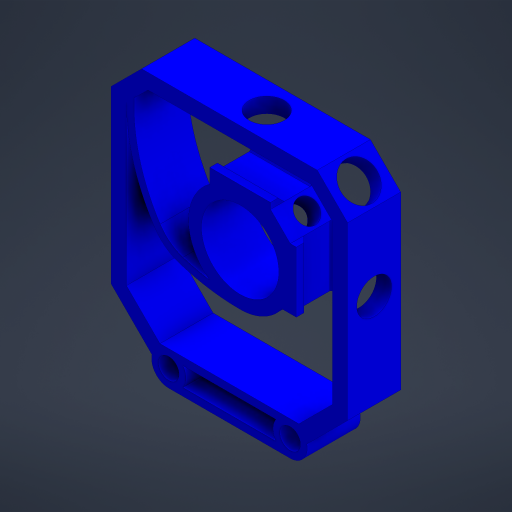
# Autodesk Inventor part: Laser Holder (Blue Laser)
Saved by Autodesk Inventor 2023.4 (Build 274418000, 418)
## iProperties
Created: 2022-07-25
Part Number: Laser Holder (Blue Laser)
Material: Generic
Document SubType Name: Modeling
Designer: xSibe
Density: 1 g/cm^3
Appearance: Plastic Blue
Author: xSibe
Autodesk Inventor part; units mm, degrees
ref_plane "YZ Plane" through (0, 0, 0) normal (1, 0, 0) x (0, 1, 0)
ref_plane "XZ Plane" through (0, 0, 0) normal (0, 1, 0) x (-1, 0, 0)
sketch "Sketch1" plane through (0, 0, 0) normal (0, 0, 1) x (1, 0, 0)
  circle A0 centre (10, 3.85) radius 1.5625
  circle A1 centre (-10, 3.85) radius 1.5625
  line L0 (-16.9, 0) -> (16.9, 0)
  line L1 (16.9, 0) -> (16.9, 7.7)
  line L2 (-16.9, 7.7) -> (16.9, 7.7)
  line L3 (-16.9, 0) -> (-16.9, 7.7)
  circle A2 centre (-10, 3.85) radius 2.8125
  circle A3 centre (10, 3.85) radius 2.8125
  line L4 (-10, 6.6625) -> (10, 6.6625)
  line L5 (10, 1.0375) -> (-10, 1.0375)
  line L6 (-10, 2.2875) -> (10, 2.2875)
  line L7 (-10, 5.4125) -> (10, 5.4125)
  line L8 (-17.05, 7.7) -> (-17.05, 42.1)
  line L9 (17.05, 7.7) -> (17.05, 42.1)
  line L10 (-17.05, 24.9) -> (17.05, 24.9)
  line L11 (0, 24.9) -> (1.767767, 26.667767)
  line L12 (0, 24.9) -> (2.5, 24.9) construction
  circle A4 centre (1.767767, 26.667767) radius 6.375
  circle A5 centre (1.767767, 26.667767) radius 5.7
  circle A6 centre (1.767767, 26.667767) radius 8.5
  line L13 (1.767767, 26.667767) -> (1.767767, 35.167767)
  line L14 (1.767767, 35.167767) -> (1.767767, 34.667767)
  line L15 (-3.232233, 33.417767) -> (6.767767, 33.417767)
  line L16 (6.767767, 33.417767) -> (6.767767, 35.917767)
  line L17 (6.767767, 35.917767) -> (-3.232233, 35.917767)
  line L18 (-3.232233, 35.917767) -> (-3.232233, 33.417767)
  line L19 (-3.232233, 33.417767) -> (6.767767, 35.917767) construction
  line L20 (6.767767, 33.417767) -> (-3.232233, 35.917767) construction
  line L21 (1.767767, 26.667767) -> (7.778175, 32.678175)
  line L22 (7.778175, 32.678175) -> (7.336233, 32.236233)
  line L23 (10.16466, 31.529126) -> (6.629126, 35.06466)
  line L24 (6.629126, 35.06466) -> (4.507806, 32.94334)
  line L25 (4.507806, 32.94334) -> (8.04334, 29.407806)
  line L26 (8.04334, 29.407806) -> (10.16466, 31.529126)
  line L27 (10.16466, 31.529126) -> (4.507806, 32.94334) construction
  line L28 (6.629126, 35.06466) -> (8.04334, 29.407806) construction
  line L29 (10.16466, 31.529126) -> (15.16466, 31.529126) construction
  line L30 (8.517767, 21.667767) -> (8.517767, 31.667767)
  line L31 (8.517767, 31.667767) -> (11.017767, 31.667767)
  line L32 (11.017767, 31.667767) -> (11.017767, 21.667767)
  line L33 (11.017767, 21.667767) -> (8.517767, 21.667767)
  line L34 (1.767767, 35.167767) -> (1.767767, 37.167767)
  line L35 (11.017767, 26.667767) -> (13.017767, 26.667767)
  line L36 (-10.217767, 5.432233) -> (10.217767, 5.432233)
  line L37 (19.467767, 14.682233) -> (19.467767, 39.367767)
  line L38 (14.467767, 44.367767) -> (-14.467767, 44.367767)
  line L39 (-19.467767, 39.367767) -> (-19.467767, 14.682233)
  line L40 (-19.467767, 5.432233) -> (19.467767, 44.367767) construction
  line L41 (19.467767, 5.432233) -> (-19.467767, 44.367767) construction
  line L42 (-10.217767, 5.432233) -> (-19.467767, 14.682233)
  line L43 (10.217767, 5.432233) -> (19.467767, 14.682233)
  line L44 (14.467767, 44.367767) -> (19.467767, 39.367767)
  line L45 (-14.467767, 44.367767) -> (-19.467767, 39.367767)
  line L46 (-15.503301, 46.867767) -> (-21.967767, 40.403301)
  line L47 (-21.967767, 40.403301) -> (-21.967767, 13.646699)
  line L48 (-21.967767, 13.646699) -> (-11.253301, 2.932233)
  line L49 (-11.253301, 2.932233) -> (11.253301, 2.932233)
  line L50 (11.253301, 2.932233) -> (21.967767, 13.646699)
  line L51 (21.967767, 13.646699) -> (21.967767, 40.403301)
  line L52 (21.967767, 40.403301) -> (15.503301, 46.867767)
  line L53 (15.503301, 46.867767) -> (-15.503301, 46.867767)
  line L54 (-13.432233, 41.867767) -> (-16.967767, 38.332233)
  line L55 (-16.967767, 38.332233) -> (-16.967767, 15.717767)
  line L56 (-16.967767, 15.717767) -> (-9.182233, 7.932233)
  line L57 (-9.182233, 7.932233) -> (9.182233, 7.932233)
  line L58 (9.182233, 7.932233) -> (16.967767, 15.717767)
  line L59 (16.967767, 15.717767) -> (16.967767, 38.332233)
  line L60 (16.967767, 38.332233) -> (13.432233, 41.867767)
  line L61 (13.432233, 41.867767) -> (-13.432233, 41.867767)
  line L62 (16.967767, 15.717767) -> (16.967767, 8.646699)
  line L63 (-16.967767, 15.717767) -> (-16.967767, 12.182233)
  line L64 (-19.467767, 14.682233) -> (-19.467767, 11.146699)
  line L65 (19.467767, 14.682233) -> (19.467767, 11.146699)
  circle A7 centre (-10, 3.85) radius 1.705
  circle A8 centre (10, 3.85) radius 1.707
  line L66 (1.767767, 18.167767) -> (-10.732233, 18.167767)
  line L67 (-10.732233, 18.167767) -> (-10.732233, 20.667767)
  arc A9 (-10.732233, 20.667767) -> (1.767767, 18.167767) centre (1.767767, 50.667767) ccw
  arc A10 (-16.967767, 38.332233) -> (-10.732233, 20.667767) centre (11.170581, 38.332233) ccw
  arc A11 (-15.687259, 39.612741) -> (-9.956996, 21.700675) centre (11.170581, 38.332233) ccw
  arc A12 (-9.956996, 21.700675) -> (-3.278671, 19.827923) centre (1.767767, 50.667767) ccw
  line L68 (-9.956996, 21.700675) -> (-11.410357, 23.734819)
  line L69 (-10.732233, 20.667767) -> (-12.213666, 22.681558)
  arc A13 (-12.213666, 22.681558) -> (-8.44317, 19.813484) centre (-6.151219, 26.73905) ccw
  arc A14 (-11.410357, 23.734819) -> (-7.660174, 20.873868) centre (-5.557613, 27.518317) ccw
  line L70 (-10, 6.6625) -> (-11.448034, 6.6625)
  line L71 (10, 6.6625) -> (11.448034, 6.6625)
  point P0 (0, 0)
  point P1 (-7.661464, 2.2875)
  point P2 (-7.661464, 5.4125)
  point P3 (7.661464, 5.4125)
  point P4 (7.661464, 2.2875)
  point P5 (7.341455, 2.932233)
  point P6 (-7.341455, 2.932233)
  point P7 (-11.185824, 6.40029)
  point P8 (11.185824, 6.40029)
  point P9 (-3.232233, 33.54163)
  point P10 (8.64163, 21.667767)
  point P11 (8.64163, 31.667767)
  point P12 (9.280097, 30.644563)
  point P13 (5.744563, 34.180097)
  point P14 (6.767767, 33.54163)
  point P15 (12.751875, 4.430808)
  point P16 (-12.751875, 4.430808)
  point P17 (4.982233, 33.417767)
  point P18 (-3.557585, 33.292767)
  point P19 (8.392767, 21.342415)
  point P20 (8.517767, 29.882233)
  point P21 (10.267767, 26.667767)
  point P22 (10.026019, 31.667767)
  point P23 (8.392767, 31.993119)
  point P24 (7.093119, 33.292767)
  point P25 (1.767767, 35.167767)
  point P26 (6.767767, 34.926019)
  point P27 (7.778175, 32.678175)
  point P28 (-17.05, 12.264466)
  point P29 (16.967767, 24.9)
  point P30 (17.05, 12.264466)
  point P31 (-16.967767, 24.9)
  point P32 (16.967767, 12.182233)
  point P33 (10.081912, 24.9)
  point P34 (-6.546378, 24.9)
  point P35 (-17.05, 41.785534)
  point P36 (17.05, 41.785534)
  point P37 (7.67477, 5.432233)
  point P38 (-7.67477, 5.432233)
  point P39 (12.485534, 7.7)
  point P40 (-12.485534, 7.7)
  point P41 (8.267767, 30.420815)
  point P42 (5.520815, 33.167767)
  dimension "d0" = 1.25
  dimension "d1" = 1.25
  dimension "d2" = 2.5
  dimension "d3" = 45
  dimension "d4" = 12.75
  dimension "d5" = 0.675
  dimension "d6" = 2.125
  dimension "d7" = 0.5
  dimension "d8" = 10
  dimension "d9" = 2.5
  dimension "d10" = 0.625
  dimension "d11" = 5
  dimension "d12" = 135
  dimension "d13" = 3
  dimension "d14" = 2
  dimension "d15" = 2
  dimension "d16" = 38.93553
  dimension "d17" = 38.93553
  dimension "d18" = 9.25
  dimension "d19" = 9.25
  dimension "d20" = 9.25
  dimension "d21" = 9.25
  dimension "d22" = 5
  dimension "d23" = 5
  dimension "d24" = 5
  dimension "d25" = 5
  dimension "d26" = 2.5
  dimension "d46" = 2.5
  dimension "d51" = 0.1425
  dimension "d52" = 0.1445
  dimension "d53" = 12.5
  dimension "d54" = 2.5
  dimension "d55" = 1.25
  dimension "d56" = 2.5
  dimension "d59" = 2.5
  constraints: 132 end point, 28 point on circle, 20 point on line, 13 centre point, 13 parallel, 13 tangent, 10 midpoint, 8 horizontal, 7 perpendicular, 4 symmetric about line, 3 vertical, 2 equal length, 1 coincident, 15 other
  measures "d0" radial gap between concentric circles of A1 A2
  measures "d1" radial gap between concentric circles of A0 A3
  measures "d2" distance of L11.start L11.end
  measures "d3" angle of L12 L11
  measures "d4" diameter of A4
  measures "d5" radial gap between concentric circles of A4 A5
  measures "d6" radial gap between concentric circles of A4 A6
  measures "d7" distance of L13.end L14.end
  measures "d8" distance of L17.end L16.end
  measures "d9" distance of L16.end L15.end
  measures "d10" distance of L21.end L22.end
  measures "d11" distance of L23.start L23.end
  measures "d12" angle of L29 L23
  measures "d13" distance of L24.end L23.end
  measures "d14" distance of L13.end L34.end
  measures "d15" distance of L35.start L35.end
  measures "d16" distance of L40.end L41.end
  measures "d17" distance of L41.end L40.start
  measures "d18" distance of L36.start L40.start
  measures "d19" distance of L39.end L40.start
  measures "d20" distance of L36.end L41.start
  measures "d21" distance of L37.start L41.start
  measures "d22" distance of L38.start L40.end
  measures "d23" distance of L37.end L40.end
  measures "d24" distance of L38.end L41.end
  measures "d25" distance of L39.start L41.end
  measures "d26" distance between parallel lines of L38 L53
  measures "d46" distance between parallel lines of L38 L61
  measures "d51" radial gap between concentric circles of A1 A7
  measures "d52" radial gap between concentric circles of A0 A8
  measures "d53" distance of L66.start L66.end
  measures "d54" distance of L66.end L67.end
  measures "d55" radial gap between concentric circles of A10 A11
  measures "d56" distance of L68.start L68.end
  measures "d59" distance of L67.end L69.end
extrude "Extrusion1" add sketch "Sketch1" along normal mid plane 8.75 contours A8 L49 A3 L7 | L7 A3 L36 A8 | A8 L43 A3 L50 | L50 A3 L6 A8 | A8 L6 A3 L49 | L7 A2 L36 A3 | L36 A3 L43 A8 | A3 L43 L2 L50 | L36 A2 L4 A3 | L7 A7 L36 A2 | A2 L49 A7 L7 | A3 L5 A2 L6 | A3 L71 L43 | L2 L43 L62 L50 | A2 L6 A7 L49 | L36 A7 L42 A2 | A2 L48 A7 L6 | L62 L43 L9 L50 | A2 L42 L70 | L42 A2 L48 L2 | L2 L48 L8 L42 | L62 L59 L10 L9 L43 | L9 L43 L65 L50 | L42 A7 L48 A2 | L42 L8 L10 L55 L63 | L9 L44 L37 L43 | L48 L64 L42 L8 | L42 L39 L45 L8 | L10 L59 L60 L61 L54 L55 L8 L45 L38 L44 L9 | L32 L33 A6 L10 | L10 A6 L26 L23 L31 L32 | A10 L54 A11 L10 | L10 A11 A12 A6 A9 A13 L69 A10 | A6 L33 L30 L10 | L10 L30 L26 A6 | L69 A13 | L30 L33 A6 L10 A4 | L10 A4 L25 L26 L30 | A6 L18 L15 L13 A4 L10 | A14 L68 A11 | L30 L31 A6 L26 | L26 L25 L21 A6 L31 L30 | A6 L31 L23 L26 | L31 A6 L16 L23 | L18 L17 L34 A6 | A6 L13 L15 L18 | L68 A14 A12 | L23 L24 A6 L34 L17 L16 | L16 A6 L24 L23 | L13 L15 L24 L25 A4 | A6 L24 L15 L13 | L25 L24 L15 L16 A6 L21 | L16 L15 L24 A6
sketch "Sketch2" plane through (0, 0, 0) normal (0, 0, 1) x (1, 0, 0)
  circle A0 centre (1.767767, 26.667767) radius 6.375
  circle A1 centre (1.767767, 26.667767) radius 5.5
  line L0 (-10, 1.0375) -> (10, 1.0375)
  arc A2 (10, 1.0375) -> (12.751875, 4.430808) centre (10, 3.85) ccw
  line L1 (12.751875, 4.430808) -> (19.467767, 11.146699)
  line L2 (19.467767, 11.146699) -> (19.467767, 39.367767)
  line L3 (19.467767, 39.367767) -> (14.467767, 44.367767)
  line L4 (14.467767, 44.367767) -> (-14.467767, 44.367767)
  line L5 (-14.467767, 44.367767) -> (-19.467767, 39.367767)
  line L6 (-19.467767, 39.367767) -> (-19.467767, 11.146699)
  line L7 (-19.467767, 11.146699) -> (-12.751875, 4.430808)
  arc A3 (-12.751875, 4.430808) -> (-10, 1.0375) centre (-10, 3.85) ccw
  line L8 (-7.661464, 5.4125) -> (7.661464, 5.4125)
  arc A4 (7.661464, 5.4125) -> (7.661464, 2.2875) centre (10, 3.85) ccw
  line L9 (7.661464, 2.2875) -> (-7.661464, 2.2875)
  arc A5 (-7.661464, 2.2875) -> (-7.661464, 5.4125) centre (-10, 3.85) ccw
  line L10 (6.767767, 35.917767) -> (-3.232233, 35.917767)
  line L11 (-3.232233, 35.917767) -> (-3.232233, 33.54163)
  line L12 (-15.687259, 39.612741) -> (-13.432233, 41.867767)
  line L13 (-13.432233, 41.867767) -> (13.432233, 41.867767)
  line L14 (13.432233, 41.867767) -> (16.967767, 38.332233)
  line L15 (16.967767, 38.332233) -> (16.967767, 12.182233)
  line L16 (16.967767, 12.182233) -> (11.448034, 6.6625)
  line L17 (-11.448034, 6.6625) -> (-16.967767, 12.182233)
  line L18 (-16.967767, 12.182233) -> (-16.967767, 38.332233)
  line L19 (8.64163, 21.667767) -> (11.017767, 21.667767)
  line L20 (11.017767, 21.667767) -> (11.017767, 31.667767)
  line L21 (11.017767, 31.667767) -> (10.026019, 31.667767)
  arc A6 (1.767767, 18.167767) -> (8.64163, 21.667767) centre (1.767767, 26.667767) ccw
  line L22 (6.767767, 34.926019) -> (6.767767, 35.917767)
  circle A7 centre (1.767767, 26.667767) radius 8.5
  line L23 (10.026019, 31.667767) -> (6.767767, 34.926019)
  arc A8 (-3.232233, 33.54163) -> (-3.278671, 19.827923) centre (1.767767, 26.667767) ccw
  arc A9 (-7.660174, 20.873868) -> (-3.278671, 19.827923) centre (1.767767, 50.667767) ccw
  arc A10 (-11.410357, 23.734819) -> (-7.660174, 20.873868) centre (-5.557613, 27.518317) ccw
  arc A11 (-15.687259, 39.612741) -> (-11.410357, 23.734819) centre (11.170581, 38.332233) ccw
  arc A12 (-16.967767, 38.332233) -> (-12.213666, 22.681558) centre (11.170581, 38.332233) ccw
  arc A13 (-12.213666, 22.681558) -> (-8.44317, 19.813484) centre (-6.151219, 26.73905) ccw
  arc A14 (-8.44317, 19.813484) -> (1.767767, 18.167767) centre (1.767767, 50.667767) ccw
  line L24 (11.448034, 6.6625) -> (-11.448034, 6.6625)
  point P0 (0, 0)
  point P1 (-4.596846, 21.033789)
  point P2 (1.767767, 18.167767)
  point P3 (5.517767, 34.29584)
  point P4 (1.767767, 35.167767)
  point P5 (9.39584, 30.417767)
  point P6 (10.267767, 26.667767)
  point P7 (8.64163, 21.667767)
  point P8 (-3.232233, 33.54163)
  dimension "d30" = 0.875
  constraints: 1 centre point, 3 other
  measures "d30" radial gap between concentric circles of A0 A1
extrude "Extrusion2" [suppressed]
sketch "Sketch3" plane through (19.467767, 13.646699, -4.375) normal (1, 0, 0) x (0, 0, -1)
  line L0 (0, 8.021068) -> (-8.75, 8.021068)
  line L1 (0, 18.021068) -> (0, 8.021068)
  line L2 (0, 18.021068) -> (-8.75, 18.021068)
  line L3 (-8.75, 8.021068) -> (-8.75, 18.021068)
  line L4 (-4.375, 18.021068) -> (-4.375, 8.021068)
  circle A0 centre (-4.375, 13.021068) radius 2.875
  point P0 (-4.375, -13.646699)
  dimension "d33" = 5.75
  constraints: 3 midpoint, 2 end point, 1 centre point
  measures "d33" diameter of A0
extrude "Extrusion3" cut sketch "Sketch3" against normal up to surface (2.5 mm away) contours A0 L4 | L4 A0
sketch "Sketch4" plane through (9.883277, 31.667767, -4.375) normal (0, 1, 0) x (1, 0, 0)
  line L0 (1.13449, 0) -> (1.13449, -8.75)
  line L1 (0.142742, 0) -> (1.13449, 0)
  line L2 (1.13449, -8.75) -> (0.142742, -8.75)
  line L3 (1.13449, -8.75) -> (0.142742, -8.75)
  line L4 (0.142742, -8.75) -> (0.142742, -7.5)
  line L5 (0.142742, -7.5) -> (1.13449, -7.5)
  line L6 (1.13449, -7.5) -> (1.13449, -8.75)
  line L7 (1.13449, -7.5) -> (0.142742, -6.508252)
  line L8 (1.13449, -7.5) -> (2.537033, -7.5) construction
  line L9 (0.142742, -4.375) -> (1.13449, -4.375)
  line L10 (1.13449, -1.25) -> (0.142742, -2.241748)
  line L11 (0.142742, 0) -> (0.142742, -8.75)
  point P0 (-9.883277, -4.375)
  point P1 (1.13449, -1.25)
  point P2 (1.13449, -7.5)
  point P3 (1.13449, -7.5)
  point P4 (0.142742, -2.241748)
  dimension "d36" = 1.25
  dimension "d37" = 135
  constraints: 16 end point, 2 horizontal, 2 midpoint, 2 parallel, 2 point on line, 2 symmetric about line, 1 equal length, 1 perpendicular
  measures "d36" distance of L3.end L4.end
  measures "d37" angle of L8 L7
extrude "Extrusion4" cut sketch "Sketch4" against normal up to surface (10 mm away) contours L0 L9 L11 L10 | L0 L7 L11 L9
ref_plane "Work Plane1" through (11.017767, 35.917767, 4.375) normal (0.7071068, -0.7071068, 0) x (0, 0, -1)
mirror "Mirror1" about plane through (11.017767, 35.917767, 4.375) normal (0.7071068, -0.7071068, 0) of "Extrusion3", "Extrusion4"
sketch "Sketch5" plane through (20.2, 38.635534, 4.375) normal (0.7071068, 0.7071068, 0) x (0.7071068, -0.7071068, 0)
  circle A0 centre (-4.571068, 4.375) radius 1.875
  line L0 (-8.106602, 4.375) -> (-1.035534, 4.375)
  circle A1 centre (-4.571068, 4.375) radius 3
  line L1 (-8.106602, 8.75) -> (-8.106602, 0)
  line L2 (-1.035534, 0) -> (-8.106602, 0)
  line L3 (-1.035534, 8.75) -> (-1.035534, 0)
  line L4 (-8.106602, 8.75) -> (-1.035534, 8.75)
  point P0 (13.035891, 4.375)
  dimension "d40" = 3.75
  dimension "d41" = 6
  constraints: 3 midpoint, 2 centre point, 2 end point, 1 coincident
  measures "d40" diameter of A0
  measures "d41" diameter of A1
extrude "Extrusion5" cut sketch "Sketch5" against normal blind 5 contours L0 A0 | L0 A1 A0 | A0 L0 A1 | A0 L0
extrude "Extrusion6" cut sketch "Sketch5" against normal up to next from surface at -12.121046 contours L0 A0 | A0 L0
equation "\"d19\" = d18"
equation "\"d20\" = d18"
equation "\"d21\" = d20"
equation "\"d23\" = d22"
equation "\"d24\" = d22"
equation "\"d25\" = d24"
body "Solid1"
